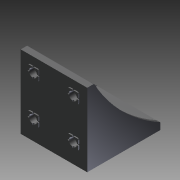
# Autodesk Inventor part: HBLFSDD6_
Saved by Autodesk Inventor 2011 SP1 (Build 150282100, 282)
## iProperties
Created: 2018-01-07
Part Number: HBLFSDD6_
Catalog Web Link: www.cadenas.de
Description: HBLFSN6, HBLFSNB6, HBLFSNM6, HBLFSNK6, HBLFSSW6, HBLFSSWB6, HBLFSSW6-50, HBLFSDW6, HBLFSDW6-50, HBLFSN6, HBLFSD6-50-Thin Reversal Brackets for Slot Width 8 Frames - For 30, 50, 60mm Sections
Vendor: MISUMI
Document SubType Name: Modeling
Designer: psAdmin
Manufacturer: MISUMI
Mass: 30.2154 g
Surface Area: 164.19 cm^2
Volume: 30.2154 cm^3
Density: 1 g/cm^3
Category: PARTsolutions
Company: MISUMI
Title: HBLFSDD6_
Author: Cadenas PARTsolutions
Comments: Thin Reversal Brackets for Slot Width 8 Frames - For 30, 50, 60mm Sections
PSOL_IDENT_0: {$CADENAS_DATA\23d-libs\misumi\metric\38_al_extrusions_blackets\6\hblfsn6.prj},279 {VTYP=3D},{NB=HBL
PSOL_IDENT_1: FSDD6_},{LINA=HBLFSDD6_},{NN=HBLFSN6, HBLFSNB6, HBLFSNM6, HBLFSNK6, HBLFSSW6, HBLFSSWB6, HBLFSSW6-50
PSOL_IDENT_2: , HBLFSDW6, HBLFSDW6-50, HBLFSN6, HBLFSD6-50},{DATE=24.04.2017 10:22:35},{GEOMDATE=09.11.2010 09:07:
PSOL_IDENT_3: 00},{VERSION=},{LINEID=310},{LINESUBID=-1},{WBVAR=ALT1,ALT2}  {NB=HBLFSDD6_},{LINA=HBLFSDD6_},{KT=8}
PSOL_IDENT_4: ,{PN=HBLFSDD6},{TP=HBLFSDD6},{NOH=2},{NOHV=2},{MAT=ADC12},{ST=-},{TYPE=HBLFSDD6},{FEAT=Reversal Brac
PSOL_IDENT_5: ket with Protrusion},{ALT1=},{ALT2=},{MASS=65},{AB=CBM6-12},{NOB=8},{AN=HNTT6-6},{NON=8},{AL=2940},{
PSOL_IDENT_6: W=50},{H=55},{DP=55},{T=5.0},{HDIS=30},{DPOS=12},{HH1=15},{HV1=25},{DIA=6.2},{ALT1OPT='','w/o C (Mou
PSOL_IDENT_7: nting Holes for Cover)','-C','with C (Mounting Holes for Cover)'},{ALT2OPT= '' , 'w/o Set Applicable
PSOL_IDENT_8: Bolt & Nut' , '-SET' , 'with SET (Set Applicable Bolt & Nut)' , '-SST' , 'with SST (Stainless Steel
PSOL_IDENT_9: Set Applicable Bolt & Nut)' , '-SEP' , 'with SEP (Post Assembly Spring Nuts Set Applicable Bolt & N
PSOL_IDENT_10: ut)' , '-SSP' , 'with SSP (Post Assembly Spring Nuts, Stainless Steel Set Applicable Bolt & Nut)'},{
PSOL_IDENT_11: R=1},{R1=0.3},{APOSV=0},{VER=1},{PR=8},{TT=0.8},{T1=5}
NN: HBLFSN6, HBLFSNB6, HBLFSNM6, HBLFSNK6, HBLFSSW6, HBLFSSWB6, HBLFSSW6-50, HBLFSDW6, HBLFSDW6-50, HBLFSN6, HBLFSD6-50
NT: Thin Reversal Brackets for Slot Width 8 Frames - For 30, 50, 60mm Sections
NB: HBLFSDD6_
NBSYN: $PN._
LINA: HBLFSDD6_
PN: HBLFSDD6
TP: HBLFSDD6
MAT: ADC12
ST: -
FEAT: Reversal Bracket with Protrusion
ALT1: w/o C (Mounting Holes for Cover)
ALT2: w/o Set Applicable Bolt & Nut
MASS: 65
AB: CBM6-12
NOB: 8
AN: HNTT6-6
NON: 8
AL: 2940
SUPPLIER: MISUMI
ARTICLENO: HBLFSDD6_
BOMINFO: HBLFSDD6_
CREATOR: CADENAS GmbH
Autodesk Inventor part; units mm, degrees
sketch "Sketch_15" plane through (0, 0, 0) normal (1, 0, 0) x (0, 1, 0)
  line L0 (4.5858, 55) -> (0, 55)
  line L1 (0, 55) -> (0, 0)
  line L2 (0, 0) -> (55, 0)
  line L3 (55, 0) -> (55, 4.5858)
  arc A0 (55, 4.5858) -> (54.7071, 5.2929) centre (54, 4.5858) ccw
  line L4 (54.7071, 5.2929) -> (5.2929, 54.7071)
  arc A1 (5.2929, 54.7071) -> (4.5858, 55) centre (4.5858, 54) ccw
  constraints: 10 end point, 4 point on circle, 2 centre point
extrude "Extrusion1" add sketch "Sketch_15" along normal mid plane 50
sketch "Sketch_16" plane through (0, 0, 0) normal (1, 0, 0) x (0, 1, 0)
  line L0 (60, 60) -> (5, 60)
  line L1 (5, 60) -> (5, 5)
  line L2 (5, 5) -> (60, 5)
  line L3 (60, 5) -> (60, 60)
  constraints: 8 end point
extrude "Extrusion2" cut sketch "Sketch_16" along normal mid plane 45
sketch "Sketch_28" plane through (0, 0, 0) normal (1, 0, 0) x (0, 1, 0)
  arc A0 (5.2929, 54.7071) -> (54.7071, 5.2929) centre (114.5616, 114.5616) ccw
  line L0 (54.7071, 5.2929) -> (5.2929, 54.7071)
  constraints: 2 end point, 2 point on circle, 1 centre point
extrude "Extrusion3" cut sketch "Sketch_28" along normal mid plane 50
sketch "Sketch_22_ALT_Drilling_1" plane through (0, 0, 0) normal (0, 1, 0) x (-1, 0, 0)
  circle A0 centre (15, 15) radius 3.1
  constraints: 1 centre point
extrude "Extrusion4" cut sketch "Sketch_22_ALT_Drilling_1" along normal blind 5
sketch "Pattern_3_SKETCH_1" plane through (30, 0, 0) normal (0, 1, 0) x (1, 0, 0)
  circle A0 centre (-15, -15) radius 3.1
  constraints: 1 centre point
sketch "Pattern_3_SKETCH_2" plane through (0, 0, 30) normal (0, 1, 0) x (1, 0, 0)
  circle A0 centre (-15, -15) radius 3.1
  constraints: 1 centre point
sketch "Pattern_3_SKETCH_3" plane through (30, 0, 30) normal (0, 1, 0) x (1, 0, 0)
  circle A0 centre (-15, -15) radius 3.1
  constraints: 1 centre point
extrude "Extrusion5" cut sketch "Pattern_3_SKETCH_1" along normal blind 5
extrude "Extrusion6" cut sketch "Pattern_3_SKETCH_2" along normal blind 5
extrude "Extrusion7" cut sketch "Pattern_3_SKETCH_3" along normal blind 5
sketch "Sketch_24_ALT_Drilling_2" plane through (0, 0, 0) normal (0, 0, 1) x (1, 0, 0)
  circle A0 centre (-15, 20) radius 3.1
  constraints: 1 centre point
extrude "Extrusion8" cut sketch "Sketch_24_ALT_Drilling_2" along normal blind 5
sketch "Pattern_4_SKETCH_1" plane through (30, 0, 0) normal (0, 0, 1) x (1, 0, 0)
  circle A0 centre (-15, 20) radius 3.1
  constraints: 1 centre point
sketch "Pattern_4_SKETCH_2" plane through (0, 25, 0) normal (0, 0, 1) x (1, 0, 0)
  circle A0 centre (-15, 20) radius 3.1
  constraints: 1 centre point
sketch "Pattern_4_SKETCH_3" plane through (30, 25, 0) normal (0, 0, 1) x (1, 0, 0)
  circle A0 centre (-15, 20) radius 3.1
  constraints: 1 centre point
extrude "Extrusion9" cut sketch "Pattern_4_SKETCH_1" along normal blind 5
extrude "Extrusion10" cut sketch "Pattern_4_SKETCH_2" along normal blind 5
extrude "Extrusion11" cut sketch "Pattern_4_SKETCH_3" along normal blind 5
sketch "Sketch_1" plane through (0, 0, 0) normal (0, 1, 0) x (-1, 0, 0)
  line L0 (25, 55) -> (-25, 55)
  line L1 (-25, 55) -> (-25, 0)
  line L2 (-25, 0) -> (25, 0)
  line L3 (25, 0) -> (25, 55)
  constraints: 8 end point
extrude "Extrusion12" add sketch "Sketch_1" against normal blind 0.8
sketch "Sketch_14" plane through (0, 0, 0) normal (0, 1, 0) x (-1, 0, 0)
  line L0 (25, 55) -> (-25, 55)
  line L1 (-25, 55) -> (-25, 0)
  line L2 (-25, 0) -> (25, 0)
  line L3 (25, 0) -> (25, 55)
  line L4 (-15.5, 18.0594) -> (-15.5, 19)
  line L5 (-15.5, 19) -> (-18, 19)
  arc A0 (-18, 19) -> (-19, 18) centre (-18, 18) ccw
  line L6 (-19, 18) -> (-19, 15.5)
  line L7 (-19, 15.5) -> (-18.0594, 15.5)
  arc A1 (-15.5, 18.0594) -> (-18.0594, 15.5) centre (-15, 15) ccw
  line L8 (-15.5, 48.0594) -> (-15.5, 49)
  line L9 (-15.5, 49) -> (-18, 49)
  arc A2 (-18, 49) -> (-19, 48) centre (-18, 48) ccw
  line L10 (-19, 48) -> (-19, 45.5)
  line L11 (-19, 45.5) -> (-18.0594, 45.5)
  arc A3 (-15.5, 48.0594) -> (-18.0594, 45.5) centre (-15, 45) ccw
  arc A4 (-18.0594, 14.5) -> (-15.5, 11.9406) centre (-15, 15) ccw
  line L12 (-18.0594, 14.5) -> (-19, 14.5)
  line L13 (-19, 14.5) -> (-19, 12)
  arc A5 (-19, 12) -> (-18, 11) centre (-18, 12) ccw
  line L14 (-18, 11) -> (-15.5, 11)
  line L15 (-15.5, 11) -> (-15.5, 11.9406)
  arc A6 (-18.0594, 44.5) -> (-15.5, 41.9406) centre (-15, 45) ccw
  line L16 (-18.0594, 44.5) -> (-19, 44.5)
  line L17 (-19, 44.5) -> (-19, 42)
  arc A7 (-19, 42) -> (-18, 41) centre (-18, 42) ccw
  line L18 (-18, 41) -> (-15.5, 41)
  line L19 (-15.5, 41) -> (-15.5, 41.9406)
  line L20 (-11, 12) -> (-11, 14.5)
  line L21 (-11, 14.5) -> (-11.9406, 14.5)
  arc A8 (-14.5, 11.9406) -> (-11.9406, 14.5) centre (-15, 15) ccw
  line L22 (-14.5, 11.9406) -> (-14.5, 11)
  line L23 (-14.5, 11) -> (-12, 11)
  arc A9 (-12, 11) -> (-11, 12) centre (-12, 12) ccw
  line L24 (-11, 15.5) -> (-11, 18)
  arc A10 (-11, 18) -> (-12, 19) centre (-12, 18) ccw
  line L25 (-12, 19) -> (-14.5, 19)
  line L26 (-14.5, 19) -> (-14.5, 18.0594)
  arc A11 (-11.9406, 15.5) -> (-14.5, 18.0594) centre (-15, 15) ccw
  line L27 (-11.9406, 15.5) -> (-11, 15.5)
  line L28 (-11, 42) -> (-11, 44.5)
  line L29 (-11, 44.5) -> (-11.9406, 44.5)
  arc A12 (-14.5, 41.9406) -> (-11.9406, 44.5) centre (-15, 45) ccw
  line L30 (-14.5, 41.9406) -> (-14.5, 41)
  line L31 (-14.5, 41) -> (-12, 41)
  arc A13 (-12, 41) -> (-11, 42) centre (-12, 42) ccw
  line L32 (-11, 45.5) -> (-11, 48)
  arc A14 (-11, 48) -> (-12, 49) centre (-12, 48) ccw
  line L33 (-12, 49) -> (-14.5, 49)
  line L34 (-14.5, 49) -> (-14.5, 48.0594)
  arc A15 (-11.9406, 45.5) -> (-14.5, 48.0594) centre (-15, 45) ccw
  line L35 (-11.9406, 45.5) -> (-11, 45.5)
  line L36 (14.5, 18.0594) -> (14.5, 19)
  line L37 (14.5, 19) -> (12, 19)
  arc A16 (12, 19) -> (11, 18) centre (12, 18) ccw
  line L38 (11, 18) -> (11, 15.5)
  line L39 (11, 15.5) -> (11.9406, 15.5)
  arc A17 (14.5, 18.0594) -> (11.9406, 15.5) centre (15, 15) ccw
  line L40 (14.5, 48.0594) -> (14.5, 49)
  line L41 (14.5, 49) -> (12, 49)
  arc A18 (12, 49) -> (11, 48) centre (12, 48) ccw
  line L42 (11, 48) -> (11, 45.5)
  line L43 (11, 45.5) -> (11.9406, 45.5)
  arc A19 (14.5, 48.0594) -> (11.9406, 45.5) centre (15, 45) ccw
  arc A20 (11.9406, 14.5) -> (14.5, 11.9406) centre (15, 15) ccw
  line L44 (11.9406, 14.5) -> (11, 14.5)
  line L45 (11, 14.5) -> (11, 12)
  arc A21 (11, 12) -> (12, 11) centre (12, 12) ccw
  line L46 (12, 11) -> (14.5, 11)
  line L47 (14.5, 11) -> (14.5, 11.9406)
  arc A22 (11.9406, 44.5) -> (14.5, 41.9406) centre (15, 45) ccw
  line L48 (11.9406, 44.5) -> (11, 44.5)
  line L49 (11, 44.5) -> (11, 42)
  arc A23 (11, 42) -> (12, 41) centre (12, 42) ccw
  line L50 (12, 41) -> (14.5, 41)
  line L51 (14.5, 41) -> (14.5, 41.9406)
  line L52 (19, 12) -> (19, 14.5)
  line L53 (19, 14.5) -> (18.0594, 14.5)
  arc A24 (15.5, 11.9406) -> (18.0594, 14.5) centre (15, 15) ccw
  line L54 (15.5, 11.9406) -> (15.5, 11)
  line L55 (15.5, 11) -> (18, 11)
  arc A25 (18, 11) -> (19, 12) centre (18, 12) ccw
  line L56 (19, 15.5) -> (19, 18)
  arc A26 (19, 18) -> (18, 19) centre (18, 18) ccw
  line L57 (18, 19) -> (15.5, 19)
  line L58 (15.5, 19) -> (15.5, 18.0594)
  arc A27 (18.0594, 15.5) -> (15.5, 18.0594) centre (15, 15) ccw
  line L59 (18.0594, 15.5) -> (19, 15.5)
  line L60 (19, 42) -> (19, 44.5)
  line L61 (19, 44.5) -> (18.0594, 44.5)
  arc A28 (15.5, 41.9406) -> (18.0594, 44.5) centre (15, 45) ccw
  line L62 (15.5, 41.9406) -> (15.5, 41)
  line L63 (15.5, 41) -> (18, 41)
  arc A29 (18, 41) -> (19, 42) centre (18, 42) ccw
  line L64 (19, 45.5) -> (19, 48)
  arc A30 (19, 48) -> (18, 49) centre (18, 48) ccw
  line L65 (18, 49) -> (15.5, 49)
  line L66 (15.5, 49) -> (15.5, 48.0594)
  arc A31 (18.0594, 45.5) -> (15.5, 48.0594) centre (15, 45) ccw
  line L67 (18.0594, 45.5) -> (19, 45.5)
  constraints: 136 end point, 64 point on circle, 32 centre point
extrude "Extrusion13" cut sketch "Sketch_14" against normal blind 0.8
ref_plane "SD6_50_1_XY" through (-10, 15, 5) normal (0, 0, 1) x (1, 0, 0)
ref_plane "SD6_50_1_YZ" through (-10, 15, 5) normal (1, 0, 0) x (0, 1, 0)
ref_plane "SD6_50_1_ZX" through (-10, 15, 5) normal (0, 1, 0) x (0, 0, 1)
ref_plane "SD6_50_2_XY" through (10, 15, 5) normal (0, 0, 1) x (1, 0, 0)
ref_plane "SD6_50_2_YZ" through (10, 15, 5) normal (1, 0, 0) x (0, 1, 0)
ref_plane "SD6_50_2_ZX" through (10, 15, 5) normal (0, 1, 0) x (0, 0, 1)
ref_plane "SD6_50_3_XY" through (-10, 5, 18) normal (0, 1, 0) x (1, 0, 0)
ref_plane "SD6_50_3_YZ" through (-10, 5, 18) normal (1, 0, 0) x (0, 0, -1)
ref_plane "SD6_50_3_ZX" through (-10, 5, 18) normal (0, 0, -1) x (0, 1, 0)
ref_plane "SD6_50_4_XY" through (10, 5, 18) normal (0, 1, 0) x (1, 0, 0)
ref_plane "SD6_50_4_YZ" through (10, 5, 18) normal (1, 0, 0) x (0, 0, -1)
ref_plane "SD6_50_4_ZX" through (10, 5, 18) normal (0, 0, -1) x (0, 1, 0)
ref_plane "a10_to_bolt_XY" through (15, 15, 5) normal (0, 0, 1) x (1, 0, 0)
ref_plane "a10_to_bolt_YZ" through (15, 15, 5) normal (1, 0, 0) x (0, 1, 0)
ref_plane "a10_to_bolt_ZX" through (15, 15, 5) normal (0, 1, 0) x (0, 0, 1)
ref_plane "a11_to_bolt_XY" through (-15, 5, 18) normal (0, 1, 0) x (1, 0, 0)
ref_plane "a11_to_bolt_YZ" through (-15, 5, 18) normal (1, 0, 0) x (0, 0, -1)
ref_plane "a11_to_bolt_ZX" through (-15, 5, 18) normal (0, 0, -1) x (0, 1, 0)
ref_plane "a12_to_bolt_XY" through (15, 5, 18) normal (0, 1, 0) x (1, 0, 0)
ref_plane "a12_to_bolt_YZ" through (15, 5, 18) normal (1, 0, 0) x (0, 0, -1)
ref_plane "a12_to_bolt_ZX" through (15, 5, 18) normal (0, 0, -1) x (0, 1, 0)
ref_plane "a13_to_bolt_XY" through (0, 5, 35) normal (0, 1, 0) x (1, 0, 0)
ref_plane "a13_to_bolt_YZ" through (0, 5, 35) normal (1, 0, 0) x (0, 0, -1)
ref_plane "a13_to_bolt_ZX" through (0, 5, 35) normal (0, 0, -1) x (0, 1, 0)
ref_plane "a14_to_bolt_XY" through (0, 40, 5) normal (0, 0, 1) x (1, 0, 0)
ref_plane "a14_to_bolt_YZ" through (0, 40, 5) normal (1, 0, 0) x (0, 1, 0)
ref_plane "a14_to_bolt_ZX" through (0, 40, 5) normal (0, 1, 0) x (0, 0, 1)
ref_plane "a1_to_bolt_XY" through (-15, 20, 5) normal (0, 0, 1) x (1, 0, 0)
ref_plane "a1_to_bolt_YZ" through (-15, 20, 5) normal (1, 0, 0) x (0, 1, 0)
ref_plane "a1_to_bolt_ZX" through (-15, 20, 5) normal (0, 1, 0) x (0, 0, 1)
ref_plane "a2_to_bolt_XY" through (-15, 5, 15) normal (0, 1, 0) x (1, 0, 0)
ref_plane "a2_to_bolt_YZ" through (-15, 5, 15) normal (1, 0, 0) x (0, 0, -1)
ref_plane "a2_to_bolt_ZX" through (-15, 5, 15) normal (0, 0, -1) x (0, 1, 0)
ref_plane "a3_to_bolt_XY" through (1, 25, 5) normal (0, 0, 1) x (1, 0, 0)
ref_plane "a3_to_bolt_YZ" through (1, 25, 5) normal (1, 0, 0) x (0, 1, 0)
ref_plane "a3_to_bolt_ZX" through (1, 25, 5) normal (0, 1, 0) x (0, 0, 1)
ref_plane "a4_to_bolt_XY" through (1, 5, 15) normal (0, 1, 0) x (1, 0, 0)
ref_plane "a4_to_bolt_YZ" through (1, 5, 15) normal (1, 0, 0) x (0, 0, -1)
ref_plane "a4_to_bolt_ZX" through (1, 5, 15) normal (0, 0, -1) x (0, 1, 0)
ref_plane "a55_to_bolt_XY" through (0, 28, 5) normal (0, 0, 1) x (1, 0, 0)
ref_plane "a55_to_bolt_YZ" through (0, 28, 5) normal (1, 0, 0) x (0, 1, 0)
ref_plane "a55_to_bolt_ZX" through (0, 28, 5) normal (0, 1, 0) x (0, 0, 1)
ref_plane "a5_to_bolt_XY" through (0, 25, 5) normal (0, 0, 1) x (1, 0, 0)
ref_plane "a5_to_bolt_YZ" through (0, 25, 5) normal (1, 0, 0) x (0, 1, 0)
ref_plane "a5_to_bolt_ZX" through (0, 25, 5) normal (0, 1, 0) x (0, 0, 1)
ref_plane "a6_to_bolt_XY" through (0, 5, 15) normal (0, 1, 0) x (1, 0, 0)
ref_plane "a6_to_bolt_YZ" through (0, 5, 15) normal (1, 0, 0) x (0, 0, -1)
ref_plane "a6_to_bolt_ZX" through (0, 5, 15) normal (0, 0, -1) x (0, 1, 0)
ref_plane "a7_to_bolt_XY" through (0, 45, 5) normal (0, 0, 1) x (1, 0, 0)
ref_plane "a7_to_bolt_YZ" through (0, 45, 5) normal (1, 0, 0) x (0, 1, 0)
ref_plane "a7_to_bolt_ZX" through (0, 45, 5) normal (0, 1, 0) x (0, 0, 1)
ref_plane "a8_to_bolt_XY" through (0, 5, 45) normal (0, 1, 0) x (1, 0, 0)
ref_plane "a8_to_bolt_YZ" through (0, 5, 45) normal (1, 0, 0) x (0, 0, -1)
ref_plane "a8_to_bolt_ZX" through (0, 5, 45) normal (0, 0, -1) x (0, 1, 0)
ref_plane "a9_to_bolt_XY" through (-15, 15, 5) normal (0, 0, 1) x (1, 0, 0)
ref_plane "a9_to_bolt_YZ" through (-15, 15, 5) normal (1, 0, 0) x (0, 1, 0)
ref_plane "a9_to_bolt_ZX" through (-15, 15, 5) normal (0, 1, 0) x (0, 0, 1)
ref_plane "bracket_to_dummy_XY" through (0, 0, 0) normal (0, 1, 0) x (1, 0, 0)
ref_plane "bracket_to_dummy_YZ" through (0, 0, 0) normal (1, 0, 0) x (0, 0, -1)
ref_plane "bracket_to_dummy_ZX" through (0, 0, 0) normal (0, 0, -1) x (0, 1, 0)
ref_plane "hole_x1_bolt_XY" through (-15, 45, 5) normal (0, 0, 1) x (1, 0, 0)
ref_plane "hole_x1_bolt_YZ" through (-15, 45, 5) normal (1, 0, 0) x (0, 1, 0)
ref_plane "hole_x1_bolt_ZX" through (-15, 45, 5) normal (0, 1, 0) x (0, 0, 1)
ref_plane "holex2_to_bolt_XY" through (15, 45, 5) normal (0, 0, 1) x (1, 0, 0)
ref_plane "holex2_to_bolt_YZ" through (15, 45, 5) normal (1, 0, 0) x (0, 1, 0)
ref_plane "holex2_to_bolt_ZX" through (15, 45, 5) normal (0, 1, 0) x (0, 0, 1)
ref_plane "holex3_to_bolt_XY" through (15, 5, 45) normal (0, 1, 0) x (1, 0, 0)
ref_plane "holex3_to_bolt_YZ" through (15, 5, 45) normal (1, 0, 0) x (0, 0, -1)
ref_plane "holex3_to_bolt_ZX" through (15, 5, 45) normal (0, 0, -1) x (0, 1, 0)
ref_plane "holex4_to_bolt_XY" through (15, 5, 15) normal (0, 1, 0) x (1, 0, 0)
ref_plane "holex4_to_bolt_YZ" through (15, 5, 15) normal (1, 0, 0) x (0, 0, -1)
ref_plane "holex4_to_bolt_ZX" through (15, 5, 15) normal (0, 0, -1) x (0, 1, 0)
ref_plane "holex5_to_bolt_XY" through (-15, 5, 45) normal (0, 1, 0) x (1, 0, 0)
ref_plane "holex5_to_bolt_YZ" through (-15, 5, 45) normal (1, 0, 0) x (0, 0, -1)
ref_plane "holex5_to_bolt_ZX" through (-15, 5, 45) normal (0, 0, -1) x (0, 1, 0)
ref_plane "holex6_to_bolt_XY" through (15, 20, 5) normal (0, 0, 1) x (1, 0, 0)
ref_plane "holex6_to_bolt_YZ" through (15, 20, 5) normal (1, 0, 0) x (0, 1, 0)
ref_plane "holex6_to_bolt_ZX" through (15, 20, 5) normal (0, 1, 0) x (0, 0, 1)
body "Solid1"
